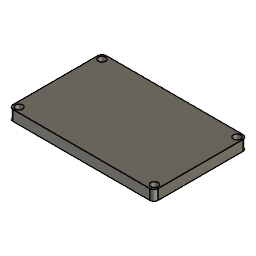
top (Autodesk Fusion 360 design; units mm, degrees)
part number: 2025-12-27-14-56-15-252
Autodesk Fusion 360 part; units mm, degrees
sketch "Sketch1" plane through (0, 0, 0) normal (0, 0, 1) x (1, 0, 0)
  line L0 (0, 0) -> (70, 0)
  line L1 (70, 0) -> (70, 45)
  line L2 (70, 45) -> (0, 45)
  line L3 (0, 45) -> (0, 0)
  circle A0 centre (2.5, 42.5) radius 1.75
  circle A1 centre (67.5, 42.5) radius 1.75
  circle A2 centre (67.5, 2.7406) radius 1.75
  circle A3 centre (2.5, 2.5) radius 1.75
  dimension "d1" = 45
  dimension "d2" = 70
  dimension "d3" = 3.5
  dimension "d4" = 3.5
  dimension "d5" = 3.5
  dimension "d6" = 3.5
  constraint horizontal L0
  constraint vertical L1
  constraint horizontal L2
  constraint vertical L3
  constraint coincident L0.start L3.end
  measures "d1" distance of L0.start L2.end
  measures "d2" distance of L1.end L2.end
  measures "d3" diameter of A1
  measures "d4" diameter of A3
  measures "d5" diameter of A0
  measures "d6" diameter of A2
extrude "Extrude1" add sketch "Sketch1" along normal blind 5
fillet "Fillet1" radius 2 4 edges at (0, 45, 2.5) (0, 0, 2.5) (70, 45, 2.5) (70, 0, 2.5)
